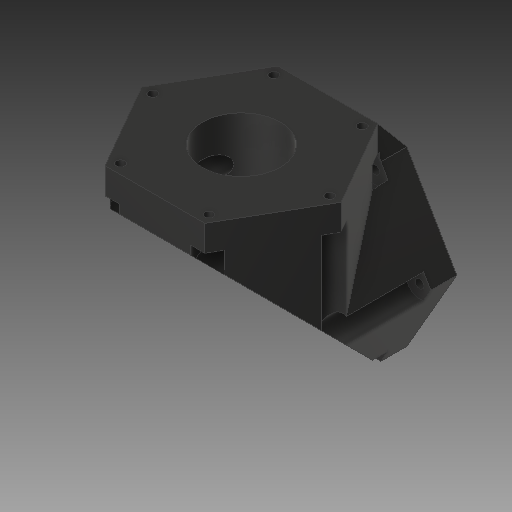
# Autodesk Inventor part: TARM14
Saved by Autodesk Inventor 2017 (Build 210142000, 142)
## iProperties
Created: 2019-01-08
Part Number: TARM14
Material: ABS Plastic
Document SubType Name: Modeling
Designer: Dell
Density: 1.06 g/cm^3
Appearance: Smooth - Black
Author: Dell
Autodesk Inventor part; units mm, degrees
ref_plane "YZ Plane" through (0, 0, 0) normal (1, 0, 0) x (0, 1, 0)
sketch "Sketch1" plane through (0, 0, 0) normal (0, 0, 1) x (1, 0, 0)
  line L0 (57.5, 0) -> (28.75, -49.7965)
  line L1 (28.75, -49.7965) -> (-28.75, -49.7965)
  line L2 (-28.75, -49.7965) -> (-57.5, 0)
  line L3 (-57.5, 0) -> (-28.75, 49.7965)
  line L4 (-28.75, 49.7965) -> (28.75, 49.7965)
  line L5 (28.75, 49.7965) -> (57.5, 0)
  circle A0 centre (0, 0) radius 22.5
  circle A1 centre (51, 0) radius 2.5
  circle A2 centre (25.5, 44.1673) radius 2.5
  circle A3 centre (-25.5, 44.1673) radius 2.5
  circle A4 centre (-51, 0) radius 2.5
  circle A5 centre (-25.5, -44.1673) radius 2.5
  circle A6 centre (25.5, -44.1673) radius 2.5
  dimension "d0" = 115
  dimension "d1" = 45
  dimension "d2" = 5
  dimension "d3" = 51
  dimension "d6" = 360
  constraints: 12 end point, 7 centre point, 2 coincident, 2 horizontal alignment, 26 other
  measures "d0" distance of L0.start L2.end
  measures "d1" diameter of A0
  measures "d2" diameter of A1
  measures "d3" distance of A1.centre point (0, 0)
extrude "Extrusion1" add sketch "Sketch1" along normal blind 15
sketch "Sketch2" plane through (-28.75, 49.7965, 0) normal (0, 1, 0) x (1, 0, 0)
  line L0 (-28.75, -66.6673) -> (0, -16.8708)
  line L1 (0, -16.8708) -> (57.5, -16.8708)
  line L2 (57.5, -16.8708) -> (86.25, -66.6673)
  line L3 (86.25, -66.6673) -> (57.5, -116.4638)
  line L4 (57.5, -116.4638) -> (0, -116.4638)
  line L5 (0, -116.4638) -> (-28.75, -66.6673)
  line L6 (0, 0) -> (57.5, 0) projected
  line L7 (0, 0) -> (-28.75, 0) projected
  line L8 (57.5, -16.8708) -> (0, -16.8708)
  line L9 (0, -16.8708) -> (0, 0)
  line L10 (0, 0) -> (57.5, 0)
  line L11 (57.5, 0) -> (57.5, -16.8708)
  circle A0 centre (28.75, -66.6673) radius 22.5
  circle A1 centre (-22.25, -66.6673) radius 2.5
  circle A2 centre (3.25, -110.8346) radius 2.5
  circle A3 centre (54.25, -110.8346) radius 2.5
  circle A4 centre (79.75, -66.6673) radius 2.5
  circle A5 centre (54.25, -22.5) radius 2.5
  circle A6 centre (3.25, -22.5) radius 2.5
  line L12 (57.5, -15) -> (0, -15) projected
  point P0 (28.75, 0)
  point P1 (28.75, 0)
  dimension "d10" = 45
  dimension "d11" = 5
  dimension "d12" = 51
  dimension "d15" = 360
  dimension "d17" = 1.8708
  constraints: 20 end point, 7 centre point, 3 vertical alignment, 2 horizontal, 2 parallel, 1 coincident, 1 horizontal alignment, 1 midpoint, 1 perpendicular, 26 other
  measures "d10" diameter of A0
  measures "d11" diameter of A1
  measures "d12" distance of A1.centre point (28.75, -66.667)
  measures "d17" distance between parallel lines of L12 L8
extrude "Extrusion2" add sketch "Sketch2" along normal blind 20
sketch "Sketch3" plane through (-28.75, 49.7965, 0) normal (0, -1, 0) x (1, 0, 0)
  line L0 (57.5, 15) -> (0, 15) projected
  line L1 (57.5, 16.8708) -> (57.5, 15) projected
  line L2 (86.25, 66.6673) -> (57.5, 16.8708) projected
  line L3 (57.5, 116.4638) -> (86.25, 66.6673) projected
  line L4 (0, 116.4638) -> (57.5, 116.4638) projected
  line L5 (-28.75, 66.6673) -> (0, 116.4638) projected
  line L6 (0, 16.8708) -> (-28.75, 66.6673) projected
  line L7 (0, 15) -> (0, 16.8708) projected
  circle A0 centre (28.75, 66.6673) radius 22.5 projected
  circle A1 centre (3.25, 22.5) radius 2.5 projected
  circle A2 centre (54.25, 22.5) radius 2.5 projected
  circle A3 centre (79.75, 66.6673) radius 2.5 projected
  circle A4 centre (54.25, 110.8346) radius 2.5 projected
  circle A5 centre (3.25, 110.8346) radius 2.5 projected
  circle A6 centre (-22.25, 66.6673) radius 2.5 projected
  circle A7 centre (79.75, 66.6673) radius 2.5 projected
  circle A8 centre (79.75, 66.6673) radius 7.5
  circle A9 centre (54.25, 110.8346) radius 7.5
  circle A10 centre (3.25, 110.8346) radius 7.5
  circle A11 centre (-22.25, 66.6673) radius 7.5
  circle A12 centre (3.25, 22.5) radius 7.5
  circle A13 centre (54.25, 22.5) radius 7.5
  point P0 (28.75, 0)
  dimension "d20" = 15
  dimension "d23" = 360
  constraints: 6 centre point, 1 coincident, 13 other
  measures "d20" diameter of A8
extrude "Extrusion3" add sketch "Sketch3" along normal blind 99.5929 contours L0 A13 L1 | L0 A12 L6 A11 L5 A10 L4 A9 L3 A8 L2 A13 | A13 L2 L1 | L0 L7 A12 | A12 L7 L6 | A8 L3 L2 | L6 L5 A11 | A9 L4 L3 | L5 L4 A10 picked at (58.5222, 20.7288) picked at (-1.0222, 20.7288) picked at (83.3394, 63.7458) picked at (-25.8394, 63.7458) picked at (53.5809, 115.4147) picked at (3.9191, 115.4147)
sketch "Sketch4" plane through (0, 0, 15) normal (0, 0, 1) x (1, 0, 0)
  circle A0 centre (0, 0) radius 22.5 projected
  circle A1 centre (25.5, -44.1673) radius 2.5 projected
  circle A2 centre (-25.5, -44.1673) radius 2.5 projected
  circle A3 centre (-51, 0) radius 2.5 projected
  circle A4 centre (-25.5, 44.1673) radius 2.5 projected
  circle A5 centre (25.5, 44.1673) radius 2.5 projected
  circle A6 centre (51, 0) radius 2.5 projected
  line L0 (57.5, 0) -> (28.75, -49.7965) projected
  line L1 (28.75, -49.7965) -> (-28.75, -49.7965) projected
  line L2 (-28.75, -49.7965) -> (-57.5, 0) projected
  line L3 (-57.5, 0) -> (-28.75, 49.7965) projected
  line L4 (-28.75, 49.7965) -> (-28.75, 69.7965) projected
  line L5 (28.75, 69.7965) -> (-28.75, 69.7965) projected
  line L6 (28.75, 49.7965) -> (28.75, 69.7965) projected
  line L7 (28.75, 49.7965) -> (57.5, 0) projected
  line L8 (-28.75, 49.7965) -> (28.75, 49.7965)
  constraints: 2 end point, 1 horizontal
extrude "Extrusion4" add sketch "Sketch4" along normal blind 104.5929 contours L0 L1 L2 L3 L8 L7
sketch "Sketch5" plane through (28.75, 49.7965, 0) normal (1, 0, 0) x (0, 0, -1)
  line L0 (-116.4638, 0) -> (-66.6673, -49.7965) projected
  line L1 (-16.8708, -99.5929) -> (-66.6673, -49.7965) projected
  line L2 (-16.8708, -99.5929) -> (-66.6673, -49.7965) projected
  line L3 (-66.6673, -99.5929) -> (-66.6673, -49.7965) projected
  line L4 (-16.8708, -99.5929) -> (-66.6673, -99.5929) projected
  line L5 (-66.6673, -49.7965) -> (-116.4638, -99.5929) projected
  line L6 (-66.6673, -99.5929) -> (-116.4638, -99.5929) projected
  line L7 (-66.6673, -99.5929) -> (-66.6673, -49.7965) projected
  line L8 (-66.6673, -49.7965) -> (-116.4638, -99.5929) projected
  line L9 (-66.6673, -49.7965) -> (-119.5929, -49.7965) projected
  line L10 (-119.5929, -99.5929) -> (-119.5929, -49.7965) projected
  line L11 (-116.4638, 0) -> (-66.6673, -49.7965) projected
  line L12 (-119.5929, -49.7965) -> (-119.5929, 0) projected
  line L13 (-66.6673, -49.7965) -> (-119.5929, -49.7965) projected
  line L14 (-116.4638, 0) -> (-119.5929, 0) projected
  line L15 (-116.4638, -99.5929) -> (-119.5929, -99.5929) projected
  point P0 (0, -49.7965)
  constraints: 1 other
extrude "Extrusion5" cut sketch "Sketch5" along normal through all both and the other way through all
sketch "Sketch6" plane through (0, 0, 0) normal (0, 0, -1) x (-1, 0, 0)
  circle A0 centre (0, 0) radius 22.5 projected
extrude "Extrusion6" cut sketch "Sketch6" against normal through all
sketch "Sketch7" plane through (-28.75, 69.7965, 0) normal (0, 1, 0) x (1, 0, 0)
  circle A0 centre (28.75, -66.6673) radius 22.5 projected
  point P0 (28.75, 0)
extrude "Extrusion7" cut sketch "Sketch7" against normal through all
fillet "Fillet1" radius 15 2 edges at (-15.9099, 15.9099, 50.7574) (15.9099, 15.9099, 50.7574)
ref_plane "Work Plane1" through (-28.75, 54.7965, 0) normal (0, 1, 0) x (1, 0, 0)
sketch "Sketch8" plane through (-28.75, 54.7965, 0) normal (0, 1, 0) x (1, 0, 0)
  arc A0 (77.25, -66.6673) -> (82.25, -66.6673) centre (79.75, -66.6673) ccw projected
  arc A1 (82.25, -66.6673) -> (77.25, -66.6673) centre (79.75, -66.6673) ccw projected
  circle A2 centre (79.75, -66.6673) radius 7.5
  circle A3 centre (28.75, -66.6673) radius 22.5 projected
  circle A4 centre (54.25, -22.5) radius 7.5
  circle A5 centre (3.25, -22.5) radius 7.5
  circle A6 centre (-22.25, -66.6673) radius 7.5
  circle A7 centre (3.25, -110.8346) radius 7.5
  circle A8 centre (54.25, -110.8346) radius 7.5
  point P0 (28.75, 0)
  dimension "d37" = 15
  dimension "d40" = 360
  constraints: 6 centre point, 1 coincident, 13 other
  measures "d37" diameter of A2
extrude "Extrusion8" cut sketch "Sketch8" against normal through all contours A1 A0 | A2 | A3 | A4 | A5 | A6 | A7 | A8
ref_plane "Work Plane2" through (0, 0, 15) normal (0, 0, -1) x (-1, 0, 0)
sketch "Sketch9" plane through (0, 0, 15) normal (0, 0, -1) x (-1, 0, 0)
  circle A0 centre (51, 0) radius 2.5 projected
  circle A1 centre (51, 0) radius 7.5
  circle A2 centre (25.5, 44.1673) radius 7.5
  circle A3 centre (-25.5, 44.1673) radius 7.5
  circle A4 centre (-51, 0) radius 7.5
  circle A5 centre (-25.5, -44.1673) radius 7.5
  circle A6 centre (25.5, -44.1673) radius 7.5
  point P0 (0, 0)
  dimension "d45" = 15
  dimension "d48" = 360
  constraints: 6 centre point, 1 coincident, 13 other
  measures "d45" diameter of A1
extrude "Extrusion9" cut sketch "Sketch9" against normal through all contours A0 | A1 | A2 | A3 | A4 | A5 | A6
sketch "Sketch10" plane through (-20.5439, 49.7965, 116.4638) normal (0, -0.7071068, 0.7071068) x (1, 0, 0)
  ellipse E0 centre (20.5439, -70.4228) end of major axis (20.5439, -102.2426) minor radius 22.5 (43.0439, -70.4228) -> (-1.9561, -70.4228) ccw projected
  ellipse E1 centre (20.5439, -70.4228) end of major axis (20.5439, -102.2426) minor radius 22.5 (-1.9561, -70.4228) -> (43.0439, -70.4228) ccw projected
  spline S0 degree 5 poles (-11.956, -70.4228) (-11.956, -70.1174) (-11.9539, -69.812) (-11.9497, -69.5066) (-11.8616, -65.2756) (-11.3663, -61.0558) (-10.5544, -57.1928) (-8.2451, -49.7983) (-4.4574, -43.0445) (-2.2338, -39.9489) (2.9623, -34.4185) (9.5234, -30.618) (13.0861, -29.2729) (20.5439, -27.9333) (28.0018, -29.2729) (31.5645, -30.618) (38.1256, -34.4185) (43.3217, -39.9489) (45.5453, -43.0445) (49.333, -49.7983) (51.6423, -57.1928) (52.4542, -61.0558) (52.9494, -65.2756) (53.0376, -69.5066) (53.0418, -69.812) (53.0439, -70.1174) (53.0439, -70.4228) knots 0 0 0 0 0 0 0.013011 0.013011 0.013011 0.180275 0.180275 0.180275 0.341166 0.341166 0.341166 0.5 0.5 0.5 0.658834 0.658834 0.658834 0.819725 0.819725 0.819725 0.986989 0.986989 0.986989 1 1 1 1 1 1
  spline S1 degree 5 poles (53.0439, -70.4228) (53.0439, -70.7283) (53.0418, -71.0337) (53.0376, -71.3391) (52.9494, -75.57) (52.4542, -79.7898) (51.6423, -83.6529) (49.333, -91.0474) (45.5453, -97.8012) (43.3217, -100.8968) (38.1256, -106.4271) (31.5645, -110.2277) (28.0018, -111.5728) (20.5439, -112.9124) (13.0861, -111.5728) (9.5234, -110.2277) (2.9623, -106.4271) (-2.2338, -100.8968) (-4.4574, -97.8012) (-8.2451, -91.0474) (-10.5544, -83.6529) (-11.3663, -79.7898) (-11.8616, -75.57) (-11.9497, -71.3391) (-11.9539, -71.0337) (-11.956, -70.7283) (-11.956, -70.4228) knots 0 0 0 0 0 0 0.013011 0.013011 0.013011 0.180275 0.180275 0.180275 0.341166 0.341166 0.341166 0.5 0.5 0.5 0.658834 0.658834 0.658834 0.819725 0.819725 0.819725 0.986989 0.986989 0.986989 1 1 1 1 1 1
  point P0 (20.5439, -117.5637)
  dimension "d52" = 10
  constraints: 2 horizontal alignment, 6 other
extrude "Extrusion10" add sketch "Sketch10" against normal blind 5 contours E1 E0 | S0 S1
sketch "Sketch12" plane through (28.75, 49.7965, 0) normal (1, 0, 0) x (0, 0, -1)
  line L0 (0, 0) -> (0, 20) projected
  line L1 (-16.8708, 20) -> (0, 20) projected
  line L2 (0, -49.7965) -> (0, 0) projected
  line L3 (-16.8708, 20) -> (-66.6673, 20) projected
  line L4 (0, 0) -> (-16.8708, 20)
  constraints: 2 end point
extrude "Extrusion11" cut sketch "Sketch12" against normal through all
body "Solid1"
